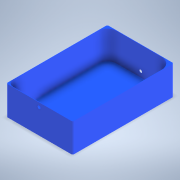
# Autodesk Inventor part: Ammonia Filter Tub
Saved by Autodesk Inventor 2020 (Build 240168000, 168)
## iProperties
Created: 2020-08-04
Part Number: Ammonia Filter Tub
Material: Generic
Document SubType Name: Modeling
Designer: Abbas
Density: 1 g/cm^3
Appearance: Default
Author: Abbas
Autodesk Inventor part; units mm, degrees
ref_plane "YZ Plane" through (0, 0, 0) normal (1, 0, 0) x (0, 1, 0)
ref_plane "XZ Plane" through (0, 0, 0) normal (0, 1, 0) x (-1, 0, 0)
ref_plane "XY Plane" through (0, 0, 0) normal (0, 0, 1) x (1, 0, 0)
sketch "Sketch1" plane through (0, 0, 0) normal (0, 1, 0) x (-1, 0, 0)
  line L0 (230, 350) -> (-230, 350)
  line L1 (-230, 350) -> (-230, -350)
  line L2 (-230, -350) -> (230, -350)
  line L3 (230, -350) -> (230, 350)
  line L4 (230, 350) -> (-230, -350) construction
  line L5 (-230, 350) -> (230, -350) construction
  line L6 (227, 347) -> (-227, 347)
  line L7 (-227, 347) -> (-227, -347)
  line L8 (-227, -347) -> (227, -347)
  line L9 (227, -347) -> (227, 347)
  line L10 (227, 347) -> (-227, -347) construction
  line L11 (-227, 347) -> (227, -347) construction
  point P0 (0, 0)
  dimension "d0" = 460
  dimension "d1" = 700
  dimension "d2" = 454
  dimension "d3" = 694
  constraints: 24 end point, 4 midpoint, 4 parallel, 2 horizontal, 2 perpendicular
  measures "d0" distance of L2.end L1.end
  measures "d1" distance of L1.end L0.end
  measures "d2" distance of L8.end L7.end
  measures "d3" distance of L7.end L6.end
extrude "Extrusion1" add sketch "Sketch1" along normal blind 3 contours L9 L8 L7 L6
extrude "Extrusion2" add sketch "Sketch1" along normal blind 200
sketch "Sketch2" plane through (-230, 0, 350) normal (0, 0, 1) x (1, 0, 0)
  line L0 (0, 0) -> (460, 0) projected
  line L1 (0, 0) -> (0, 200) projected
  point P0 (230, 0)
  point P1 (227, 170)
  dimension "d15" = 170
  dimension "d16" = 227
  measures "d15" distance from line of point (227, 170) L0
  measures "d16" distance from line of L1 point (227, 170)
hole "Hole1" at (-3, 170, 350) direction (0, 0, -1) diameter 20 depth 3 tip angle 118
sketch "Sketch3" plane through (230, 0, -350) normal (0, 0, -1) x (-1, 0, 0)
  line L0 (0, 0) -> (0, 200) projected
  line L1 (0, 0) -> (460, 0) projected
  point P0 (230, 0)
  point P1 (227, 40)
  dimension "d24" = 227
  dimension "d25" = 40
  measures "d24" distance from line of L0 point (227, 40)
  measures "d25" distance from line of L1 point (227, 40)
hole "Hole2" at (3, 40, -350) direction (0, 0, 1) diameter 20 depth 3 tip angle 118
fillet "Fillet1" radius 10 4 edges at (230, 100, 350) (230, 100, -350) (-230, 100, 350) (-230, 100, -350)
fillet "Fillet2" radius 41.7 1 edges at (-227, 101.5, 347)
fillet "Fillet3" radius 63.3 1 edges at (-227, 101.5, -347)
fillet "Fillet4" radius 78.1 1 edges at (227, 101.5, -347)
fillet "Fillet5" radius 43.7 1 edges at (227, 101.5, 347)
body "Solid1"
